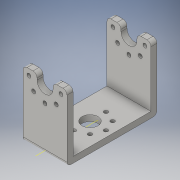
# Autodesk Inventor part: Down_Part_Robot
Saved by Autodesk Inventor 2016 (Build 200138000, 138)
## iProperties
Created: 2015-09-24
Part Number: Down_Part_Robot
Material: Generic
Document SubType Name: Modeling
Designer: fei
Density: 1 g/cm^3
Appearance: Default
Author: fei
Autodesk Inventor part; units mm, degrees
ref_plane "YZ Plane" through (0, 0, 0) normal (1, 0, 0) x (0, 1, 0)
ref_plane "XZ Plane" through (0, 0, 0) normal (0, 1, 0) x (-1, 0, 0)
ref_plane "XY Plane" through (0, 0, 0) normal (0, 0, 1) x (1, 0, 0)
sketch "Sketch1" plane through (0, 0, 0) normal (0, 0, 1) x (1, 0, 0)
  line L0 (-279.4, 38.1) -> (279.4, 38.1)
  line L1 (279.4, 38.1) -> (279.4, -38.1)
  line L2 (279.4, -38.1) -> (-279.4, -38.1)
  line L3 (-279.4, -38.1) -> (-279.4, 38.1)
  line L4 (0, 0) -> (0, 412.8984) construction
  line L5 (0, 0) -> (748.8943, 0) construction
  dimension "d0" = 558.8
  dimension "d1" = 76.2
  dimension "d2" = 38.1
  dimension "d4" = 279.4
  constraints: 12 end point, 3 parallel, 1 horizontal, 1 perpendicular, 1 vertical
  measures "d0" distance of L1.end L2.end
  measures "d1" distance of L0.end L1.end
  measures "d2" distance between parallel lines of L5 L0
  measures "d4" distance between parallel lines of L4 L1
extrude "Extrusion1" add sketch "Sketch1" along normal mid plane 1143
sketch "Sketch2" plane through (-279.4, 38.1, 571.5) normal (0, 1, 0) x (1, 0, 0)
  line L0 (558.8, 0) -> (558.8, 1143) projected
  line L1 (0, 1143) -> (0, 0) projected
  line L2 (558.8, 1143) -> (0, 1143)
  line L3 (0, 1143) -> (0, 1066.8)
  line L4 (0, 1066.8) -> (558.8, 1066.8)
  line L5 (558.8, 1066.8) -> (558.8, 1143)
  point P0 (279.4, 571.5)
  dimension "d7" = 76.2
  constraints: 8 end point, 2 parallel, 1 horizontal, 1 perpendicular, 1 point on line
  measures "d7" distance of L0.end L4.end
extrude "Extrusion2" add sketch "Sketch2" along normal blind 762
mirror "Mirror1" about plane through (0, 0, 0) normal (0, 0, 1) of "Extrusion2"
sketch "Sketch3" plane through (-279.4, 38.1, -495.3) normal (0, 1, 0) x (1, 0, 0)
  circle A0 centre (279.4, -495.3) radius 101.6
  circle A1 centre (279.4, -292.1) radius 25.4
  line L0 (558.8, -990.6) -> (558.8, 0) projected
  circle A2 centre (423.0841, -351.6159) radius 25.4
  circle A3 centre (482.6, -495.3) radius 25.4
  circle A4 centre (423.0841, -638.9841) radius 25.4
  circle A5 centre (279.4, -698.5) radius 25.4
  dimension "d10" = 203.2
  dimension "d11" = 50.8
  dimension "d12" = 203.2
  dimension "d13" = 279.4
  dimension "d16" = 180
  constraints: 6 centre point, 1 coincident, 9 other
  measures "d10" diameter of A0
  measures "d11" diameter of A1
  measures "d12" distance of A1.centre point (279.4, -495.3)
  measures "d13" distance from line of L0 A1.centre
extrude "Extrusion3" cut sketch "Sketch3" against normal through all
sketch "Sketch4" plane through (0, 0, -571.5) normal (0, 0, -1) x (-1, 0, 0)
  line L0 (-314.4934, 723.9) -> (334.7896, 723.9) construction
  line L1 (279.4, 800.1) -> (-279.4, 800.1) construction
  arc A0 (-101.6, 723.9) -> (101.6, 723.9) centre (0, 723.9) ccw
  line L2 (279.4, -38.1) -> (279.4, 800.1) projected
  line L3 (-279.4, 800.1) -> (279.4, 800.1) projected
  line L4 (101.6, 723.9) -> (101.6, 800.1)
  line L5 (-101.6, 723.9) -> (-101.6, 800.1)
  circle A1 centre (-203.2, 723.9) radius 25.4
  circle A2 centre (-143.6841, 580.2159) radius 25.4
  circle A3 centre (0, 520.7) radius 25.4
  circle A4 centre (143.6841, 580.2159) radius 25.4
  circle A5 centre (203.2, 723.9) radius 25.4
  point P0 (0, 0)
  dimension "d20" = 76.2
  dimension "d21" = 203.2
  dimension "d22" = 279.4
  dimension "d23" = 50.8
  dimension "d24" = 203.2
  dimension "d27" = 180
  constraints: 6 centre point, 6 end point, 6 point on line, 2 perpendicular, 2 point on circle, 2 tangent, 1 horizontal, 9 other
  measures "d20" distance between parallel lines of L1 L0
  measures "d21" diameter of A0
  measures "d22" distance from line of L2 A0.centre
  measures "d23" diameter of A1
  measures "d24" distance of A1.centre A0.centre
extrude "Extrusion4" cut sketch "Sketch4" against normal through all
fillet "Fillet1" radius 50.8 10 edges at (101.6, 800.1, -533.4) (-101.6, 800.1, -533.4) (-101.6, 800.1, 533.4) (101.6, 800.1, 533.4) (279.4, 800.1, 533.4) (-279.4, 800.1, 533.4) (279.4, 800.1, -533.4) (-279.4, 800.1, -533.4) (0, -38.1, -571.5) (0, -38.1, 571.5)
body "Solid1"
